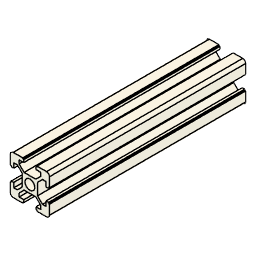
_2020 Extrusion.d20cdcef-b238-4049-98ed-29df6a03594f (Autodesk Fusion 360 design; units mm, degrees)
Autodesk Fusion 360 part; units mm, degrees
sketch "Sketch1" plane through (0, 0, 0) normal (0, 0, 1) x (1, 0, 0)
  circle A0 centre (10, 10) radius 2.5
  line L0 (13.9, 6.1) -> (6.1, 13.9) construction
  line L1 (0, 6.4) -> (0, 1.5)
  line L2 (4.5, 1.8) -> (6.9, 1.8)
  line L3 (3.5808, 4.5) -> (6.1, 7.0192)
  line L4 (4.5, 3.5808) -> (7.0192, 6.1)
  line L5 (0.5, 6.9) -> (0.5, 6.4)
  line L6 (0.5, 6.4) -> (0, 6.4)
  line L7 (6.9, 0) -> (6.4, 0) construction
  line L8 (6.4, 0) -> (6.4, 0.5)
  line L9 (6.4, 0.5) -> (6.9, 0.5)
  arc A1 (0, 1.5) -> (1.5, 0) centre (1.5, 1.5) ccw
  line L10 (1.8, 6.9) -> (0.5, 6.9)
  line L11 (1.8, 6.9) -> (1.8, 6.4)
  line L12 (1.8, 6.4) -> (1.8, 4.5)
  line L13 (3.5808, 4.5) -> (1.8, 4.5)
  line L14 (6.1, 10) -> (6.1, 7.0192)
  line L15 (7.0192, 6.1) -> (10, 6.1)
  line L16 (4.5, 1.8) -> (4.5, 3.5808)
  line L17 (6.9, 0.5) -> (6.9, 1.8)
  line L18 (1.5, 0) -> (6.4, 0)
  line L19 (6.4, 0) -> (6.9, 0)
  line L20 (0, 6.9) -> (0, 6.4)
  line L21 (10, 13.9) -> (10, 6.1) construction
  line L22 (13.9, 10) -> (6.1, 10) construction
  line L23 (20, 6.4) -> (19.5, 6.4)
  line L24 (19.5, 6.4) -> (19.5, 6.9)
  line L25 (19.5, 6.9) -> (18.2, 6.9)
  line L26 (18.2, 4.5) -> (18.2, 6.9)
  line L27 (18.2, 4.5) -> (16.4192, 4.5)
  line L28 (16.4192, 4.5) -> (13.9, 7.0192)
  line L29 (13.9, 7.0192) -> (13.9, 10)
  line L30 (15.5, 3.5808) -> (12.9808, 6.1)
  line L31 (15.5, 3.5808) -> (15.5, 1.8)
  line L32 (13.6, 1.8) -> (15.5, 1.8)
  line L33 (13.1, 1.8) -> (13.6, 1.8)
  line L34 (13.1, 1.8) -> (13.1, 0.5)
  line L35 (13.1, 0.5) -> (13.6, 0.5)
  line L36 (13.6, 0.5) -> (13.6, 0)
  line L37 (10, 6.1) -> (12.9808, 6.1)
  line L38 (13.6, 0) -> (18.5, 0)
  arc A2 (18.5, 0) -> (20, 1.5) centre (18.5, 1.5) ccw
  line L39 (20, 1.5) -> (20, 6.4)
  line L40 (13.6, 20) -> (13.6, 19.5)
  line L41 (13.6, 19.5) -> (13.1, 19.5)
  line L42 (13.1, 19.5) -> (13.1, 18.2)
  line L43 (15.5, 18.2) -> (13.1, 18.2)
  line L44 (15.5, 18.2) -> (15.5, 16.4192)
  line L45 (15.5, 16.4192) -> (12.9808, 13.9)
  line L46 (12.9808, 13.9) -> (10, 13.9)
  line L47 (16.4192, 15.5) -> (13.9, 12.9808)
  line L48 (16.4192, 15.5) -> (18.2, 15.5)
  line L49 (18.2, 13.6) -> (18.2, 15.5)
  line L50 (18.2, 13.1) -> (18.2, 13.6)
  line L51 (18.2, 13.1) -> (19.5, 13.1)
  line L52 (19.5, 13.1) -> (19.5, 13.6)
  line L53 (19.5, 13.6) -> (20, 13.6)
  line L54 (13.9, 10) -> (13.9, 12.9808)
  line L55 (20, 13.6) -> (20, 18.5)
  arc A3 (20, 18.5) -> (18.5, 20) centre (18.5, 18.5) ccw
  line L56 (18.5, 20) -> (13.6, 20)
  line L57 (0, 13.6) -> (0.5, 13.6)
  line L58 (0.5, 13.6) -> (0.5, 13.1)
  line L59 (0.5, 13.1) -> (1.8, 13.1)
  line L60 (1.8, 15.5) -> (1.8, 13.1)
  line L61 (1.8, 15.5) -> (3.5808, 15.5)
  line L62 (3.5808, 15.5) -> (6.1, 12.9808)
  line L63 (6.1, 12.9808) -> (6.1, 10)
  line L64 (4.5, 16.4192) -> (7.0192, 13.9)
  line L65 (4.5, 16.4192) -> (4.5, 18.2)
  line L66 (6.4, 18.2) -> (4.5, 18.2)
  line L67 (6.9, 18.2) -> (6.4, 18.2)
  line L68 (6.9, 18.2) -> (6.9, 19.5)
  line L69 (6.9, 19.5) -> (6.4, 19.5)
  line L70 (6.4, 19.5) -> (6.4, 20)
  line L71 (10, 13.9) -> (7.0192, 13.9)
  line L72 (6.4, 20) -> (1.5, 20)
  arc A4 (1.5, 20) -> (0, 18.5) centre (1.5, 18.5) ccw
  line L73 (0, 18.5) -> (0, 13.6)
  arc A5 (26, 1.5) -> (27.5, 0) centre (27.5, 1.5) ccw
  line L74 (41.5, 3.5808) -> (41.5, 1.8)
  line L75 (39.1, 19.5) -> (39.1, 18.2)
  line L76 (32.4, 20) -> (27.5, 20)
  line L77 (26, 6.9) -> (26, 6.4)
  line L78 (29.5808, 4.5) -> (32.1, 7.0192)
  line L79 (29.5808, 15.5) -> (32.1, 12.9808)
  line L80 (26, 13.6) -> (26.5, 13.6)
  line L81 (39.1, 0.5) -> (39.6, 0.5)
  line L82 (30.5, 16.4192) -> (30.5, 18.2)
  line L83 (27.8, 15.5) -> (27.8, 13.1)
  line L84 (36, 13.9) -> (36, 6.1) construction
  line L85 (32.4, 0) -> (32.4, 0.5)
  line L86 (39.6, 0.5) -> (39.6, 0)
  line L87 (32.1, 10) -> (32.1, 7.0192)
  line L88 (32.4, 19.5) -> (32.4, 20)
  line L89 (39.1, 1.8) -> (39.6, 1.8)
  line L90 (27.8, 6.9) -> (27.8, 6.4)
  line L91 (41.5, 16.4192) -> (38.9808, 13.9)
  line L92 (26.5, 13.1) -> (27.8, 13.1)
  line L93 (26.5, 6.4) -> (26, 6.4)
  line L94 (32.1, 12.9808) -> (32.1, 10)
  line L95 (27.5, 0) -> (32.4, 0)
  line L96 (32.9, 0.5) -> (32.9, 1.8)
  line L97 (32.9, 0) -> (32.4, 0) construction
  line L98 (30.5, 1.8) -> (30.5, 3.5808)
  line L99 (32.9, 19.5) -> (32.4, 19.5)
  line L100 (32.9, 18.2) -> (32.4, 18.2)
  line L101 (41.5, 18.2) -> (39.1, 18.2)
  line L102 (39.6, 19.5) -> (39.1, 19.5)
  line L103 (27.8, 6.9) -> (26.5, 6.9)
  line L104 (27.8, 15.5) -> (29.5808, 15.5)
  line L105 (36, 13.9) -> (33.0192, 13.9)
  line L106 (33.0192, 6.1) -> (36, 6.1)
  line L107 (41.5, 18.2) -> (41.5, 16.4192)
  line L108 (39.9, 10) -> (32.1, 10) construction
  line L109 (39.6, 1.8) -> (41.5, 1.8)
  line L110 (39.9, 6.1) -> (32.1, 13.9) construction
  line L111 (39.6, 0) -> (44.5, 0)
  line L112 (36, 6.1) -> (38.9808, 6.1)
  circle A6 centre (36, 10) radius 2.5
  line L113 (42.4192, 4.5) -> (39.9, 7.0192)
  line L114 (38.9808, 13.9) -> (36, 13.9)
  line L115 (41.5, 3.5808) -> (38.9808, 6.1)
  line L116 (39.9, 7.0192) -> (39.9, 10)
  line L117 (39.9, 10) -> (39.9, 12.9808)
  line L118 (30.5, 16.4192) -> (33.0192, 13.9)
  line L119 (42.4192, 15.5) -> (39.9, 12.9808)
  line L120 (26, 18.5) -> (26, 13.6)
  line L121 (39.6, 20) -> (39.6, 19.5)
  line L122 (32.4, 18.2) -> (30.5, 18.2)
  line L123 (26.5, 6.9) -> (26.5, 6.4)
  line L124 (39.1, 1.8) -> (39.1, 0.5)
  arc A7 (27.5, 20) -> (26, 18.5) centre (27.5, 18.5) ccw
  line L125 (44.5, 20) -> (39.6, 20)
  line L126 (26, 6.4) -> (26, 1.5)
  line L127 (30.5, 3.5808) -> (33.0192, 6.1)
  line L128 (32.4, 0) -> (32.9, 0)
  line L129 (32.4, 0.5) -> (32.9, 0.5)
  line L130 (29.5808, 4.5) -> (27.8, 4.5)
  line L131 (27.8, 6.4) -> (27.8, 4.5)
  line L132 (30.5, 1.8) -> (32.9, 1.8)
  line L133 (26.5, 13.6) -> (26.5, 13.1)
  line L134 (32.9, 18.2) -> (32.9, 19.5)
  line L135 (59.9, 6.1) -> (52.1, 13.9) construction
  circle A8 centre (56, 10) radius 2.5
  line L136 (56, 13.9) -> (56, 6.1) construction
  line L137 (66, 13.6) -> (66, 18.5)
  line L138 (61.5, 16.4192) -> (58.9808, 13.9)
  line L139 (59.9, 10) -> (59.9, 12.9808)
  line L140 (64.2, 13.1) -> (65.5, 13.1)
  line L141 (59.6, 20) -> (59.6, 19.5)
  line L142 (52.1, 12.9808) -> (52.1, 10)
  line L143 (59.1, 19.5) -> (59.1, 18.2)
  line L144 (64.2, 13.1) -> (64.2, 13.6)
  line L145 (64.2, 13.6) -> (64.2, 15.5)
  line L146 (59.9, 10) -> (52.1, 10) construction
  line L147 (65.5, 13.1) -> (65.5, 13.6)
  line L148 (64.5, 20) -> (59.6, 20)
  line L149 (49.5808, 15.5) -> (52.1, 12.9808)
  line L150 (52.4, 19.5) -> (52.4, 20)
  line L151 (62.4192, 15.5) -> (64.2, 15.5)
  line L152 (59.1, 0.5) -> (59.6, 0.5)
  line L153 (65.5, 13.6) -> (66, 13.6)
  line L154 (50.5, 16.4192) -> (53.0192, 13.9)
  line L155 (61.5, 18.2) -> (61.5, 16.4192)
  line L156 (53.0192, 6.1) -> (56, 6.1)
  line L157 (50.5, 16.4192) -> (50.5, 18.2)
  line L158 (52.4, 0.5) -> (52.9, 0.5)
  line L159 (59.1, 1.8) -> (59.6, 1.8)
  line L160 (49.5808, 4.5) -> (52.1, 7.0192)
  line L161 (50.5, 1.8) -> (50.5, 3.5808)
  line L162 (61.5, 3.5808) -> (61.5, 1.8)
  line L163 (56, 13.9) -> (53.0192, 13.9)
  line L164 (52.4, 0) -> (52.4, 0.5)
  line L165 (50.5, 3.5808) -> (53.0192, 6.1)
  line L166 (66, 1.5) -> (66, 6.4)
  line L167 (59.6, 1.8) -> (61.5, 1.8)
  arc A9 (66, 18.5) -> (64.5, 20) centre (64.5, 18.5) ccw
  line L168 (52.1, 10) -> (52.1, 7.0192)
  line L169 (64.2, 4.5) -> (62.4192, 4.5)
  line L170 (59.6, 19.5) -> (59.1, 19.5)
  line L171 (61.5, 18.2) -> (59.1, 18.2)
  line L172 (61.5, 3.5808) -> (58.9808, 6.1)
  line L173 (52.9, 0) -> (52.4, 0) construction
  line L174 (59.9, 7.0192) -> (59.9, 10)
  line L175 (52.4, 18.2) -> (50.5, 18.2)
  line L176 (59.6, 0.5) -> (59.6, 0)
  line L177 (52.9, 18.2) -> (52.4, 18.2)
  line L178 (66, 6.4) -> (65.5, 6.4)
  line L179 (56, 6.1) -> (58.9808, 6.1)
  line L180 (52.9, 18.2) -> (52.9, 19.5)
  line L181 (59.6, 0) -> (64.5, 0)
  line L182 (62.4192, 4.5) -> (59.9, 7.0192)
  arc A10 (64.5, 0) -> (66, 1.5) centre (64.5, 1.5) ccw
  line L183 (50.5, 1.8) -> (52.9, 1.8)
  line L184 (52.4, 20) -> (47.5, 20)
  line L185 (64.2, 4.5) -> (64.2, 6.9)
  line L186 (65.5, 6.4) -> (65.5, 6.9)
  line L187 (52.4, 0) -> (52.9, 0)
  line L188 (52.9, 19.5) -> (52.4, 19.5)
  line L189 (65.5, 6.9) -> (64.2, 6.9)
  line L190 (59.1, 1.8) -> (59.1, 0.5)
  line L191 (47.5, 0) -> (52.4, 0)
  line L192 (58.9808, 13.9) -> (56, 13.9)
  line L193 (62.4192, 15.5) -> (59.9, 12.9808)
  line L194 (52.9, 0.5) -> (52.9, 1.8)
  line L195 (44.5, 20) -> (47.5, 20)
  line L196 (44.5, 0) -> (47.5, 0)
  line L197 (41.5, 18.2) -> (42.8, 18.2) construction
  line L198 (42.8, 18.2) -> (49.2, 18.2)
  line L199 (49.2, 1.8) -> (42.8, 1.8)
  line L200 (42.4192, 15.5) -> (42.8, 15.8808)
  line L201 (49.5808, 15.5) -> (49.2, 15.8808)
  line L202 (49.5808, 4.5) -> (49.2, 4.1192)
  line L203 (42.4192, 4.5) -> (42.8, 4.1192)
  line L204 (42.8, 15.8808) -> (42.8, 18.2)
  line L205 (49.2, 18.2) -> (49.2, 15.8808)
  line L206 (49.2, 4.1192) -> (49.2, 1.8)
  line L207 (42.8, 1.8) -> (42.8, 4.1192)
  point P0 (10, 10)
  point P1 (36, 10)
  point P2 (56, 10)
  dimension "d3" = 5
  dimension "d6" = 6.9
  dimension "d7" = 6.9
  dimension "d14" = 6.4
  dimension "d22" = 0.5
  dimension "d23" = 0.5
  dimension "d24" = 0.5
  dimension "d25" = 0.5
  dimension "d26" = 1.5
  dimension "d28" = 360
  dimension "d30" = 360
  dimension "d31" = 5
  dimension "d32" = 0.5
  dimension "d33" = 0.5
  dimension "d34" = 0.5
  dimension "d35" = 0.5
  dimension "d36" = 1.5
  dimension "d39" = 5
  dimension "d42" = 0.5
  dimension "d43" = 0.5
  dimension "d45" = 1.3
  dimension "d47" = 6.4
  constraint horizontal L18
  constraint coincident L0 P0
  constraint coincident P0 A0.centre
  constraint vertical L1
  constraint vertical L11
  constraint horizontal L2
  constraint vertical L5
  constraint horizontal L6
  constraint horizontal L7
  constraint vertical L8
  constraint horizontal L9
  constraint tangent L1 A1
  constraint tangent A1 L18
  constraint perpendicular L15 L21
  constraint perpendicular L14 L22
  constraint horizontal L95
  constraint coincident P1 L110
  constraint coincident P1 A6.centre
  constraint vertical L126
  constraint vertical L90
  constraint horizontal L132
  constraint vertical L123
  constraint horizontal L93
  constraint horizontal L97
  constraint vertical L85
  constraint horizontal L129
  constraint tangent A5 L126
  constraint tangent A5 L95
  constraint perpendicular L84 L106
  constraint perpendicular L87 L108
  constraint horizontal L191
  constraint coincident P2 L135
  constraint coincident P2 A8.centre
  constraint horizontal L183
  constraint horizontal L173
  constraint vertical L164
  constraint horizontal L158
  constraint perpendicular L136 L156
  constraint perpendicular L146 L168
  constraint perpendicular L107 L195
  constraint parallel L191 L196
  constraint perpendicular L107 L197
  constraint horizontal L198
  constraint horizontal L199
  constraint parallel L119 L200
  constraint perpendicular L200 L201
  constraint perpendicular L201 L202
  constraint perpendicular L202 L203
  constraint vertical L204
  constraint vertical L205
  constraint vertical L206
  constraint vertical L207
  measures "d3" diameter of A0
  measures "d6" distance of origin L7.start
  measures "d7" distance of origin L20.start
  measures "d14" distance of origin L1.start
  measures "d22" distance of L20.start L5.start
  measures "d23" distance of L20.start L1.start
  measures "d24" distance of L7.start L7.end
  measures "d25" distance of L7.start L9.end
  measures "d26" radius of A1
  measures "d31" diameter of A6
  measures "d32" distance of L77.start L103.end
  measures "d33" distance of L77.start L77.end
  measures "d34" distance of L97.start L85.start
  measures "d35" distance of L97.start L96.start
  measures "d36" radius of A5
  measures "d39" diameter of A8
  measures "d42" distance of L173.start L164.start
  measures "d43" distance of L173.start L158.end
  measures "d45" distance of L101.start L197.end
  measures "d47" distance of L197.end L198.end
extrude "Extrude1" add sketch "Sketch1" along normal blind 100 makes body 1 at (12.4876, 9.7511, 33.3333) makes body 2 at (38.4876, 9.7511, 33.3333)
hidden bodies 2
equation "d7 = 10 mm - 3.1 mm"
equation "d14 = 10 mm - 3.6 mm"
named bodies: "2020 Extrusion", "2040 Extrusion"
